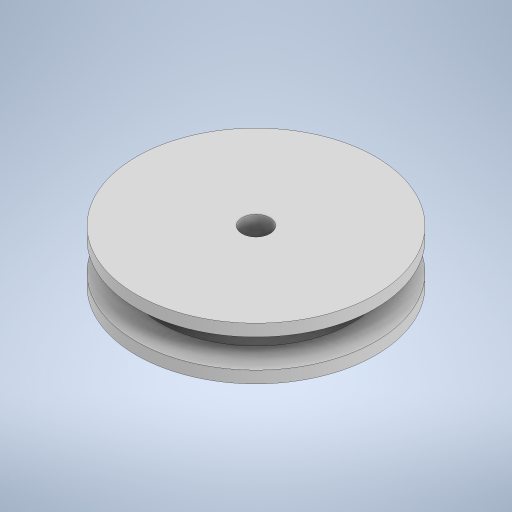
# Autodesk Inventor part: 회전 축 휠
Saved by Autodesk Inventor 2023.1 (Build 271208000, 208)
## iProperties
Created: 2022-09-04
Part Number: 회전 축 휠
Material: 일반
Document SubType Name: Modeling
Designer: fly01
Density: 1 g/cm^3
Appearance: 기본값
Author: fly01
Autodesk Inventor part; units mm, degrees
ref_plane "YZ Plane" through (0, 0, 0) normal (1, 0, 0) x (0, 1, 0)
ref_plane "XZ Plane" through (0, 0, 0) normal (0, 1, 0) x (-1, 0, 0)
ref_plane "XY Plane" through (0, 0, 0) normal (0, 0, 1) x (1, 0, 0)
sketch "스케치1" plane through (0, 0, 0) normal (0, 0, 1) x (1, 0, 0)
  line L0 (0, 0) -> (12, 0) construction
  line L1 (12, 0) -> (12, 1.3)
  line L2 (12, 1.3) -> (15, 1.8)
  line L3 (15, 1.8) -> (15, 3.3)
  line L4 (15, 3.3) -> (0, 3.3)
  line L5 (0, 3.3) -> (0, 0)
  line L6 (12, 0) -> (12, -1.3)
  line L7 (12, -1.3) -> (15, -1.8)
  line L8 (15, -1.8) -> (15, -3.3)
  line L9 (15, -3.3) -> (0, -3.3)
  line L10 (0, -3.3) -> (0, 0)
  line L11 (1.75, 3.3) -> (1.75, -3.3)
  dimension "d0" = 3.3
  dimension "d1" = 15
  dimension "d2" = 12
  dimension "d3" = 0.5
  dimension "d4" = 1.5
  dimension "d6" = 1.75
  constraints: 24 end point, 4 perpendicular, 4 symmetric about line, 2 point on line, 1 horizontal, 1 parallel
  measures "d0" distance between parallel lines of L4 L0
  measures "d1" distance of L3.end L4.end
  measures "d2" distance between parallel lines of L5 L1
  measures "d3" vertical distance of L2.end L1.end
  measures "d4" distance of L2.end L3.end
  measures "d6" distance between parallel lines of L10 L11
revolve "회전1" add sketch "스케치1" angle 360 about axis through (0, 3.3, 0) along (0, -1, 0) contours L6 L7 L8 L9 L11 L4 L3 L2 L1
